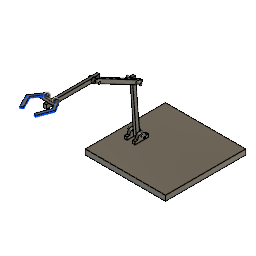
_mechanix.db008c68-67ed-4364-aed9-70695f8b2ca4 (Autodesk Fusion 360 design; units mm, degrees)
Autodesk Fusion 360 part; units mm, degrees
sketch "Sketch1" plane through (0, 0, 0) normal (0, 0, 1) x (1, 0, 0)
  line L0 (-40, 40) -> (260, 40)
  line L1 (260, 40) -> (260, -260)
  line L2 (260, -260) -> (-40, -260)
  line L3 (-40, -260) -> (-40, 40)
  dimension "d1" = 300
  dimension "d2" = 300
extrude "Extrude1" add sketch "Sketch1" along normal blind 20 makes body 1
sketch "Sketch2" plane through (0, 0, 20) normal (0, 0, 1) x (-1, 0, 0)
  line L0 (40, 260) -> (-260, 260)
  line L1 (-260, 260) -> (-260, -40)
  line L2 (-260, -40) -> (40, -40)
  line L3 (40, -40) -> (40, 260)
sketch "Sketch3" plane through (0, 0, 0) normal (1, 0, 0) x (0, 1, 0)
  line L0 (-260, 20) -> (40, 20)
  line L1 (-153.7222, 20) -> (-103.7222, 20)
  line L2 (-153.7222, 20) -> (-153.7222, 30)
  line L3 (-153.7222, 30) -> (-140, 30)
  line L4 (-140, 30) -> (-103.3, 30.3)
  line L5 (-103.3, 30.3) -> (-103.2021, 20)
  circle A0 centre (-128.0647, 30.15) radius 15.163
  circle A1 centre (-128, 36) radius 3.6056
  dimension "d5" = 50
extrude "Extrude2" add sketch "Sketch3" along normal blind 10 contours L0 L1 L4 L5 A0 | L0 L1 L3 L4 A0 | L0 L1 L2 L3 A0 | L3 L4 A0 bodies 1
sketch "Sketch4" plane through (0, 0, 0) normal (1, 0, 0) x (0, 1, 0)
ref_plane "WorkPlane1" through (30, 0, 0) normal (1, 0, 0) x (0, 1, 0)
sketch "Sketch5" plane through (30, 0, 0) normal (1, 0, 0) x (0, 1, 0)
  line L0 (-260, 20) -> (40, 20)
  line L1 (-153.7222, 20) -> (-103.2021, 20)
  line L2 (-103.3, 30.3) -> (-153.7222, 30)
  line L3 (-153.7222, 30) -> (-153.7222, 20)
  circle A0 centre (-128, 36) radius 3.6056
  arc A1 (-112.902, 30.2215) -> (-143.227, 30) centre (-128.0647, 30.15) ccw
  line L4 (-103.3, 30.3) -> (-103.2021, 20)
extrude "Extrude3" add sketch "Sketch5" along normal blind 10 bodies 1
sketch "Sketch6" plane through (40, 0, 0) normal (1, 0, 0) x (0, 1, 0)
  circle A0 centre (-128, 36) radius 3.6056
  arc A1 (-112.9021, 30.2429) -> (-143.2274, 30.0624) centre (-128.0647, 30.15) ccw
  line L0 (-143.2274, 30.0624) -> (-153.7222, 30)
  line L1 (-153.7222, 30) -> (-153.7222, 20)
  line L2 (-153.7222, 20) -> (-103.2021, 20)
  line L3 (-103.2021, 20) -> (-103.3, 30.3)
  line L4 (-103.3, 30.3) -> (-112.9021, 30.2429)
  circle A2 centre (-128, 36) radius 3.4801
extrude "Extrude4" add sketch "Sketch6" along normal blind 10 and the other way blind 50 separate body contours A2 makes body 2
sketch "Sketch7" plane through (0, 0, 0) normal (1, 0, 0) x (0, 1, 0)
  line L0 (-153.7222, 20) -> (-103.2021, 20)
  line L1 (-134, 28) -> (-121, 28)
  line L2 (-121, 28) -> (-136.2039, 227.4213)
  line L3 (-134, 28) -> (-148.9386, 226.8365)
  line L4 (-148.9386, 226.8365) -> (-136.2039, 227.4213)
  dimension "d15" = 200
extrude "Extrude5" add sketch "Sketch7" along normal blind 10 separate body makes body 3
move_body "Move1" bodies 3 to x (1, 0, 0) y (0, 1, 0) z (0, 0, 1) at (15, 0, 0)
sketch "Sketch8" plane through (25, 0, 0) normal (1, 0, 0) x (0, 1, 0)
  line L0 (-134, 28) -> (-121, 28)
  line L1 (-121, 28) -> (-136.2039, 227.4213)
  line L2 (-136.2039, 227.4213) -> (-148.9386, 226.8365)
  line L3 (-148.9386, 226.8365) -> (-134, 28)
  line L4 (-120, 210) -> (-296.7576, 303.5775)
  line L5 (-296.7576, 303.5775) -> (-303.9578, 289.9772)
  line L6 (-303.9578, 289.9772) -> (-126.64, 197.4656)
  line L7 (-126.64, 197.4656) -> (-120, 210)
  dimension "d18" = 200
extrude "Extrude6" add sketch "Sketch8" along normal blind 10 contours L3 L4 L5 L6 | L1 L3 L4 L6 | L1 L4 L6 L7 bodies 3
sketch "Sketch9" plane through (35, 0, 0) normal (1, 0, 0) x (0, 1, 0)
  line L0 (-126.64, 197.4656) -> (-120, 210)
  line L1 (-120, 210) -> (-296.7576, 303.5775)
  line L2 (-296.7576, 303.5775) -> (-303.9578, 289.9772)
  line L3 (-303.9578, 289.9772) -> (-126.64, 197.4656)
  circle A0 centre (-140.8866, 213.5255) radius 5
  dimension "d21" = 10
  measures "d21" diameter of A0
extrude "Extrude7" cut sketch "Sketch9" against normal through all contours A0 bodies 3
sketch "Sketch10" plane through (35, 0, 0) normal (1, 0, 0) x (0, 1, 0)
  circle A0 centre (-140.8866, 213.5255) radius 5
  line L0 (-126.64, 197.4656) -> (-120, 210)
  line L1 (-120, 210) -> (-296.7576, 303.5775)
  line L2 (-296.7576, 303.5775) -> (-303.9578, 289.9772)
  line L3 (-303.9578, 289.9772) -> (-126.64, 197.4656)
  circle A1 centre (-140.8866, 213.5255) radius 4.7148
extrude "Extrude8" add sketch "Sketch10" along normal blind 14 and the other way blind 37 separate body contours A1 makes body 4
sketch "Sketch11" plane through (25, 0, 0) normal (-1, 0, 0) x (0, -1, 0)
  line L0 (148.82, 225.2576) -> (147.5516, 208.3758)
  line L1 (147.5516, 208.3758) -> (303.9578, 289.9772)
  line L2 (303.9578, 289.9772) -> (296.7576, 303.5775)
  line L3 (296.7576, 303.5775) -> (148.82, 225.2576)
  line L4 (270, 300) -> (470, 300)
  line L5 (270, 300) -> (270, 285)
  line L6 (270, 285) -> (470, 285)
  line L7 (470, 285) -> (470, 300)
  dimension "d27" = 200
  measures "d27" distance of origin
extrude "Extrude9" add sketch "Sketch11" along normal blind 10 contours L3 L4 L5 | L1 L2 L3 L4 L5 L6 | L1 L2 L4 L6 L7 bodies 3
sketch "Sketch12" plane through (0, 0, 0) normal (0, 0, 1) x (1, 0, 0)
  line L0 (50, -450) -> (-10, -450)
  line L1 (-10, -450) -> (-10, -460)
  line L2 (-10, -460) -> (50, -460)
  line L3 (50, -460) -> (50, -450)
extrude "Extrude10" add sketch "Sketch12" along normal blind 10 separate body makes body 5
move_body "Move2" bodies 5 to x (1, 0, 0) y (0, 1, 0) z (0, 0, 1) at (0, 0, 300)
sketch "Sketch13" plane through (35, 0, 0) normal (1, 0, 0) x (0, 1, 0)
  circle A0 centre (-140.8866, 213.5255) radius 5
  line L0 (-126.64, 197.4656) -> (-120, 210)
  line L1 (-120, 210) -> (-296.7576, 303.5775)
  line L2 (-296.7576, 303.5775) -> (-303.9578, 289.9772)
  line L3 (-303.9578, 289.9772) -> (-126.64, 197.4656)
  circle A1 centre (-292, 292) radius 5
  dimension "d32" = 10
  measures "d32" diameter of A1
extrude "Extrude11" cut sketch "Sketch13" against normal through all contours A1 bodies 3
sketch "Sketch14" plane through (35, 0, 0) normal (1, 0, 0) x (0, 1, 0)
  circle A0 centre (-292, 292) radius 5
  circle A1 centre (-140.8866, 213.5255) radius 5
  line L0 (-126.64, 197.4656) -> (-120, 210)
  line L1 (-120, 210) -> (-296.7576, 303.5775)
  line L2 (-296.7576, 303.5775) -> (-303.9578, 289.9772)
  line L3 (-303.9578, 289.9772) -> (-126.64, 197.4656)
  circle A2 centre (-292, 292) radius 4.6816
extrude "Extrude12" add sketch "Sketch14" along normal blind 11 and the other way blind 27 separate body contours A2 makes body 6
sketch "Sketch15" plane through (0, 0, 310) normal (0, 0, 1) x (-1, 0, 0)
  line L0 (-50, 460) -> (-50, 450)
  line L1 (-50, 450) -> (10, 450)
  line L2 (10, 450) -> (10, 460)
  line L3 (10, 460) -> (-50, 460)
  line L4 (0, 445) -> (30, 490)
  line L5 (30, 490) -> (22.4663, 495.0224)
  line L6 (22.4663, 495.0224) -> (-7.5486, 450)
  line L7 (0, 445) -> (-7.5486, 450)
  line L8 (-40, 450) -> (-47.5393, 445)
  line L9 (-47.5393, 445) -> (-74.5642, 485.7499)
  line L10 (-40, 450) -> (-67.0654, 490.8111)
  line L11 (-67.0654, 490.8111) -> (-74.5642, 485.7499)
  line L12 (30, 490) -> (5, 540)
  line L13 (5, 540) -> (-5, 535)
  line L14 (-5, 535) -> (18.1935, 488.6131)
  line L15 (-62.9854, 484.6589) -> (-45, 535)
  line L16 (-45, 535) -> (-53.9927, 540)
  line L17 (-53.9927, 540) -> (-74.5642, 485.7499)
extrude "Extrude14" add sketch "Sketch15" along normal blind 5 contours L0 L1 L3 L10 | L0 L1 L3 L8 L9 L10 L11 | L3 L4 L5 L6 | L1 L3 L4 L6 | L10 L11 L15 L16 L17 | L1 L4 L7 | L5 L6 L12 L13 L14 bodies 5
extrude "Extrude13" add sketch "Sketch15" along normal blind 5 contours L0 L1 L3 L10 | L0 L1 L3 L8 L9 L10 L11 | L3 L4 L5 L6 | L1 L3 L4 L6 | L1 L4 L7 bodies 5
